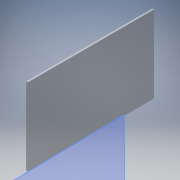
# Autodesk Inventor part: Inner side wall
Saved by Autodesk Inventor 2017 (Build 210142000, 142)
## iProperties
Created: 2017-09-30
Part Number: Inner side wall
Material: Glass
Document SubType Name: Modeling
Designer: Kenneth
Density: 2.18 g/cm^3
Appearance: Clear
Author: Kenneth
Autodesk Inventor part; units mm, degrees
ref_plane "YZ Plane" through (0, 0, 0) normal (1, 0, 0) x (0, 1, 0)
ref_plane "XZ Plane" through (0, 0, 0) normal (0, 1, 0) x (-1, 0, 0)
ref_plane "XY Plane" through (0, 0, 0) normal (0, 0, 1) x (1, 0, 0)
sketch "Sketch1" plane through (0, 0, 0) normal (1, 0, 0) x (0, 1, 0)
  line L0 (0, 0) -> (0, -457.2)
  line L1 (0, -457.2) -> (279.4, -457.2)
  line L2 (279.4, -457.2) -> (279.4, 0)
  line L3 (279.4, 0) -> (0, 0)
  dimension "d0" = 457.2
  dimension "d1" = 279.4
  constraints: 8 end point, 2 parallel, 1 perpendicular, 1 vertical
  measures "d0" distance of L1.end L2.end
  measures "d1" distance of L2.end L0.start
extrude "Extrusion1" add sketch "Sketch1" along normal blind 6.35
body "Solid1"
